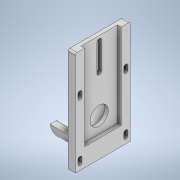
# Autodesk Inventor part: sample-transfer_slider-plate
Saved by Autodesk Inventor 2020.1 (Build 241239000, 239)
## iProperties
Created: 2019-08-16
Part Number: sample-transfer_slider-plate
Material: Generic
Document SubType Name: Modeling
Designer: rainer
Density: 1 g/cm^3
Appearance: Default
Author: rainer
Autodesk Inventor part; units mm, degrees
ref_plane "YZ Plane" through (0, 0, 0) normal (1, 0, 0) x (0, 1, 0)
ref_plane "XZ Plane" through (0, 0, 0) normal (0, 1, 0) x (-1, 0, 0)
ref_plane "XY Plane" through (0, 0, 0) normal (0, 0, 1) x (1, 0, 0)
sketch "Sketch1" plane through (0, 0, 0) normal (1, 0, 0) x (0, 1, 0)
  line L0 (25, 15) -> (-25, 15)
  line L1 (-25, 15) -> (-25, -15)
  line L2 (-25, -15) -> (25, -15)
  line L3 (25, -15) -> (25, 15)
  point P0 (0, 0)
  point P1 (25, 0)
  point P2 (0, -15)
  dimension "d0" = 30
  dimension "d1" = 50
  constraints: 8 end point, 2 midpoint, 2 parallel, 1 horizontal, 1 horizontal alignment, 1 perpendicular, 1 vertical alignment
  measures "d0" distance of L2.end L0.start
  measures "d1" distance of L1.end L2.end
extrude "Extrusion1" add sketch "Sketch1" along normal blind 2
sketch "Sketch2" plane through (2, 0, 0) normal (1, 0, 0) x (0, 0, -1)
  line L0 (-12.5, 8.5) -> (12.5, 8.5)
  line L1 (12.5, 8.5) -> (12.5, -22.5)
  line L2 (12.5, -22.5) -> (-12.5, -22.5)
  line L3 (-12.5, -22.5) -> (-12.5, 8.5)
  line L4 (-15, -25) -> (15, -25) projected
  point P0 (0, 0)
  point P1 (0, 8.5)
  dimension "d4" = 25
  dimension "d5" = 31
  dimension "d6" = 2.5
  constraints: 8 end point, 4 coincident, 2 parallel, 1 horizontal, 1 midpoint, 1 perpendicular, 1 vertical alignment
  measures "d4" distance of L0.start L0.end
  measures "d5" distance of L0.end L1.end
  measures "d6" distance between parallel lines of L4 L2
hole "Hole1" at (2, 8.5, 12.5) at (2, 8.5, -12.5) at (2, -22.5, -12.5) at (2, -22.5, 12.5) direction (-1, 0, 0) diameter 2.2 depth 5
thicken "Thicken1" operation add thickness 2 both sides no extend neighbours yes toward (1, 0, 0) faces at (2, -2.1351, -3.9584)
sketch "Sketch3" plane through (4, -25, 15) normal (1, 0, 0) x (0, 0, -1)
  line L0 (30, 50) -> (0, 50) projected
  line L1 (5, 50) -> (25, 50)
  line L2 (25, 50) -> (25, 5)
  line L3 (25, 5) -> (5, 5)
  line L4 (5, 5) -> (5, 50)
  point P0 (15, 25)
  point P1 (15, 5)
  dimension "d16" = 20
  dimension "d17" = 45
  constraints: 8 end point, 2 parallel, 1 horizontal, 1 midpoint, 1 perpendicular, 1 point on line, 1 vertical alignment
  measures "d16" distance of L2.end L3.end
  measures "d17" distance of L1.end L2.end
extrude "Extrusion2" cut sketch "Sketch3" against normal blind 2
sketch "Sketch4" plane through (0, 0, 0) normal (-1, 0, 0) x (0, 0, 1)
  circle A0 centre (0, -8.4) radius 5
  circle A1 centre (12.5, 8.5) radius 1.1 projected
  point P0 (0, 0)
  dimension "d20" = 10
  dimension "d21" = 16.9
  constraints: 1 centre point
  measures "d20" diameter of A0
  measures "d21" vertical distance of A1.centre A0.centre
extrude "Extrusion3" cut sketch "Sketch4" against normal blind 2 contours A0
sketch "Sketch5" plane through (2, -25, 15) normal (1, 0, 0) x (0, 0, -1)
  line L0 (16.25, 48) -> (13.75, 48)
  line L1 (13.75, 48) -> (13.75, 24)
  line L2 (13.75, 24) -> (16.25, 24)
  line L3 (16.25, 24) -> (16.25, 48)
  line L4 (5, 50) -> (25, 50) projected
  point P0 (15, 25)
  point P1 (15, 24)
  dimension "d24" = 24
  dimension "d25" = 2.5
  dimension "d26" = 2
  constraints: 8 end point, 2 parallel, 1 horizontal, 1 midpoint, 1 perpendicular, 1 vertical alignment
  measures "d24" distance of L2.end L0.start
  measures "d25" distance of L0.start L0.end
  measures "d26" distance between parallel lines of L4 L0
extrude "Extrusion4" cut sketch "Sketch5" against normal blind 2
thicken "Thicken2" operation add thickness 10 both sides no extend neighbours yes toward (0, 1, 0) faces at (0.6667, -1, 0.4167)
thicken "Thicken3" operation add thickness 2 both sides no extend neighbours yes toward (0, 1, 0) faces at (1.3333, 9, -0.4167)
fillet "Fillet1" radius 1 2 edges at (1, 11, 1.25) (1, 11, -1.25)
thicken "Thicken4" operation add thickness 5 both sides no extend neighbours yes toward (0, 1, 0) faces at (3.3333, -20, 3.3333)
thicken "Thicken5" operation add thickness 5 both sides no extend neighbours yes toward (0, 1, 0) faces at (0.6667, 25, -3.3333)
thicken "Thicken6" operation add thickness 5 both sides no extend neighbours yes toward (0, 1, 0) faces at (1.3333, 23, -0.4167)
fillet "Fillet2" radius 1 4 edges at (2, 30, 15) (2, 30, -15) (1, 28, 1.25) (1, 28, -1.25)
thicken "Thicken7" operation add thickness 2 both sides no extend neighbours yes toward (0, -1, 0) faces at (2.6667, -15, 3.3333)
sketch "Sketch6" plane through (0, 0, 0) normal (-1, 0, 0) x (0, 0, 1)
  circle A0 centre (0, -8.4) radius 5 projected
  circle A1 centre (0, -8.4) radius 15
  circle A2 centre (0, -8.4) radius 11
  point P0 (0, 0)
  dimension "d43" = 30
  dimension "d44" = 22
  constraints: 2 centre point, 2 coincident
  measures "d43" diameter of A1
  measures "d44" diameter of A2
extrude "Extrusion5" add sketch "Sketch6" along normal blind 10 contours A1
sketch "Sketch7" plane through (0, 0, 0) normal (-1, 0, 0) x (0, 0, 1)
  line L0 (15, -8.4) -> (15, -25) projected
  line L1 (-15, 7) -> (15, 7)
  line L2 (15, 7) -> (15, -11)
  line L3 (15, -11) -> (-15, -11)
  line L4 (-15, -11) -> (-15, 7)
  line L5 (0.25, 11) -> (-0.25, 11) projected
  point P0 (0, 0)
  dimension "d47" = 4
  dimension "d48" = 18
  dimension "d49" = 30
  constraints: 8 end point, 2 parallel, 1 horizontal, 1 perpendicular, 1 point on line
  measures "d47" distance between parallel lines of L5 L1
  measures "d48" distance of L1.end L2.end
  measures "d49" distance of L1.start L1.end
extrude "Extrusion6" cut sketch "Sketch7" along normal blind 20
fillet "Fillet3" radius 1 2 edges at (-5, -11, -10.6883) (-5, -11, 10.6883)
sketch "Sketch8" plane through (0, 0, 0) normal (-1, 0, 0) x (0, 0, 1)
  circle A0 centre (-12.5, 8.5) radius 1.1 projected
  circle A1 centre (-12.5, 9.6) radius 1.1
  circle A2 centre (-12.5, 7.4) radius 1.1
  line L0 (-13.6, 9.6) -> (-11.4, 9.6)
  line L1 (-11.4, 9.6) -> (-11.4, 7.4)
  line L2 (-11.4, 7.4) -> (-13.6, 7.4)
  line L3 (-13.6, 7.4) -> (-13.6, 9.6)
  circle A3 centre (12.5, 8.5) radius 1.1 projected
  circle A4 centre (12.5, 9.6) radius 1.1
  circle A5 centre (12.5, 7.4) radius 1.1
  line L4 (11.4, 9.6) -> (13.6, 9.6)
  line L5 (13.6, 9.6) -> (13.6, 7.4)
  line L6 (13.6, 7.4) -> (11.4, 7.4)
  line L7 (11.4, 7.4) -> (11.4, 9.6)
  circle A6 centre (12.5, -22.5) radius 1.1 projected
  circle A7 centre (12.5, -23.6) radius 1.1
  circle A8 centre (12.5, -21.4) radius 1.1
  line L8 (11.4, -21.4) -> (13.6, -21.4)
  line L9 (13.6, -21.4) -> (13.6, -23.6)
  line L10 (13.6, -23.6) -> (11.4, -23.6)
  line L11 (11.4, -23.6) -> (11.4, -21.4)
  circle A9 centre (-12.5, -22.5) radius 1.1 projected
  circle A10 centre (-12.5, -21.4) radius 1.1
  circle A11 centre (-12.5, -23.6) radius 1.1
  line L12 (-13.6, -21.4) -> (-11.4, -21.4)
  line L13 (-11.4, -21.4) -> (-11.4, -23.6)
  line L14 (-11.4, -23.6) -> (-13.6, -23.6)
  line L15 (-13.6, -23.6) -> (-13.6, -21.4)
  point P0 (0, 0)
  point P1 (-11.4, -22.5)
  point P2 (-13.6, -22.5)
  point P3 (-11.4, -21.4)
  point P4 (-13.4526, -21.95)
  point P5 (-11.5474, -21.95)
  point P6 (-11.4, 8.5)
  point P7 (-13.6, 8.5)
  point P8 (-13.6, 7.4)
  point P9 (-11.4, 9.6)
  point P10 (13.6, 8.5)
  point P11 (11.4, 8.5)
  point P12 (-13.6, 7.4)
  point P13 (-11.4, 8.4925)
  dimension "d53" = 2.2
  dimension "d54" = 2.2
  dimension "d55" = 2.2
  dimension "d56" = 2.2
  dimension "d57" = 2.2
  dimension "d58" = 2.2
  dimension "d59" = 2.2
  dimension "d60" = 2.2
  dimension "d67" = 2.2
  constraints: 32 end point, 8 parallel, 8 point on circle, 4 horizontal, 4 perpendicular, 24 other
  measures "d67" distance between parallel lines of L2 L0
extrude "Extrusion7" cut sketch "Sketch8" against normal blind 10 contours L1 A2 A0 | A0 A1 L1 | A0 L0 A1 | A2 L2 A0 | L0 A1 | A2 L2 | A0 A1 L0 | L2 A2 A0 | A1 A0 L3 | L3 A0 A2 | L5 A5 A3 | A3 A4 L5 | A3 L4 A4 | A5 L6 A3 | L4 A4 | A5 L6 | A3 A4 L4 | L6 A5 A3 | A4 A3 L7 | L7 A3 A5 | A6 A7 A8 | L9 A7 A6 | A6 A8 L9 | A8 A6 | A6 L8 A8 | A7 L10 A6 | A6 A7 | L8 A8 | A7 L10 | A6 A8 L8 | A7 A6 A8 | L10 A7 A6 | A8 A6 L11 | L11 A6 A7 | L13 A11 A9 | A9 A10 L13 | A10 A9 | A9 L12 A10 | A11 L14 A9 | L12 A10 | A11 L14 | A9 A10 L12 | L14 A11 A9 | A10 A9 L15 | L15 A9 A11
thicken "Thicken8" operation add thickness 2 both sides no extend neighbours yes toward (0, -1, 0) faces at (2.6667, -25, -5)
thicken "Thicken9" operation add thickness 0.5 both sides no extend neighbours yes toward (0, -1, 0) faces at (0.6667, 30, -3.3333)
body "Solid1"
